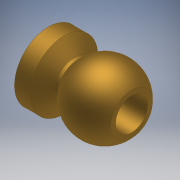
# Autodesk Inventor part: Rotule avec meplat
Saved by Autodesk Inventor 2017 (Build 210142000, 142)
## iProperties
Company: FABLAB Frenchmakers
Part Number: Rotule avec meplat
Material: Laiton, jaune doux
Document SubType Name: Modeling
Designer: FABLAB Frenchmakers
Density: 8.47 g/cm^3
Appearance: Laiton - Satiné
Mass: 1.27205 g
Surface Area: 2.7445 cm^2
Volume: 0.150182 cm^3
Project: 1420 Vauban 3D XL
Catalog Web Link: http://frenchmakers.com/
Stock Number: 1420-10-03
Autodesk Inventor part; units mm, degrees
ref_plane "YZ Plane" through (0, 0, 0) normal (1, 0, 0) x (0, 1, 0)
ref_plane "XZ Plane" through (0, 0, 0) normal (0, 1, 0) x (-1, 0, 0)
ref_plane "XY Plane" through (0, 0, 0) normal (0, 0, 1) x (1, 0, 0)
sketch "Esquisse1" plane through (0, 0, 0) normal (0, 0, 1) x (1, 0, 0)
  line L0 (-7.1186, 0) -> (5.8768, 0)
  line L1 (-4, 0) -> (-4, 3.25)
  line L2 (-4, 3.25) -> (-2.5, 3.25)
  line L3 (-2.5, 3.25) -> (-1.5, 1.95)
  line L4 (-1.5, 1.95) -> (-1.1617, 1.95)
  arc A0 (4, 2) -> (-1.1617, 1.95) centre (1.4383, 0) ccw
  line L5 (4, 2) -> (4, 0)
  line L6 (-4, 0) -> (4, 0)
  point P0 (0, 0)
  dimension "d1" = 6.5
  dimension "d2" = 8
  dimension "d3" = 1.5
  dimension "d5" = 2.5
  dimension "d6" = 4
  dimension "d7" = 6.5
  dimension "d8" = 4
  dimension "d9" = 3.9
  constraints: 14 end point, 3 horizontal, 3 perpendicular, 3 point on line, 2 point on circle, 1 centre point, 1 horizontal alignment
  measures "d1" diameter of A0
  measures "d2" distance between parallel lines of L1 L5
  measures "d3" distance of L1.end L2.end
  measures "d5" distance from line of L1 L3.end
  measures "d6" diameter of L5.start L0
  measures "d7" diameter of L2 L0
  measures "d8" distance from line of point (0, 0) L1
  measures "d9" diameter of L4 L0
revolve "Révolution1" add sketch "Esquisse1" angle 360 about axis through (-7.1186, 0, 0) along (1, 0, 0)
sketch "Esquisse2" plane through (-4, 0, 0) normal (-1, 0, 0) x (0, 0, 1)
  point P0 (0, 0)
  point P1 (0, 0)
  constraints: 1 coincident
hole "Perçage1" at (-4, 0, 0) direction (1, 0, 0) diameter 3.1 end through all countersink diameter 3.5 countersink angle 90
equation "\"d8\" = 0.5 * d2"
